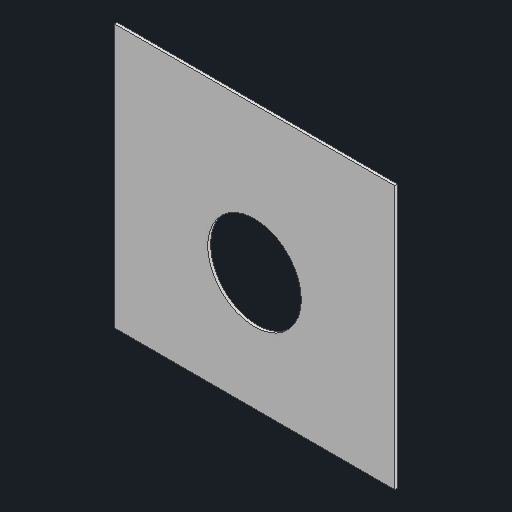
# Autodesk Inventor part: второй верх
Saved by Autodesk Inventor 2026.2 (Build 302298000, 298)
## iProperties
Created: 2025-11-21
Part Number: второй верх
Material: Типовые
Document SubType Name: Modeling
Designer: Phantom
Density: 1 g/cm^3
Appearance: По умолчанию
Author: Phantom
Autodesk Inventor part; units mm, degrees
ref_plane "YZ Plane" through (0, 0, 0) normal (1, 0, 0) x (0, 1, 0)
ref_plane "XZ Plane" through (0, 0, 0) normal (0, 1, 0) x (-1, 0, 0)
ref_plane "XY Plane" through (0, 0, 0) normal (0, 0, 1) x (1, 0, 0)
sketch "Эскиз1" plane through (0, 0, 0) normal (0, 0, 1) x (1, 0, 0)
  line L0 (-202.5, -190) -> (202.5, -190)
  line L1 (202.5, -190) -> (202.5, 190)
  line L2 (202.5, 190) -> (-202.5, 190)
  line L3 (-202.5, 190) -> (-202.5, -190)
  line L4 (-202.5, -190) -> (202.5, 190) construction
  line L5 (202.5, -190) -> (-202.5, 190) construction
  point P0 (0, 0)
  dimension "d0" = 405
  dimension "d1" = 380
  constraints: 12 end point, 2 midpoint, 2 parallel, 1 horizontal, 1 perpendicular
  measures "d0" distance of L2.end L1.end
  measures "d1" distance of L1.end L0.end
extrude "Выдавливание1" add sketch "Эскиз1" along normal blind 4
sketch "Эскиз2" plane through (0, 0, 4) normal (0, 0, 1) x (1, 0, 0)
  line L0 (-202.5, -190) -> (202.5, -190) projected
  line L1 (80, -190) -> (-80, -190)
  circle A0 centre (-0.0936, -20) radius 67.5 projected
  point P0 (0, 0)
  point P1 (0, -80)
  constraints: 2 end point, 1 point on line
extrude "Выдавливание2" cut sketch "Эскиз2" against normal blind 10
